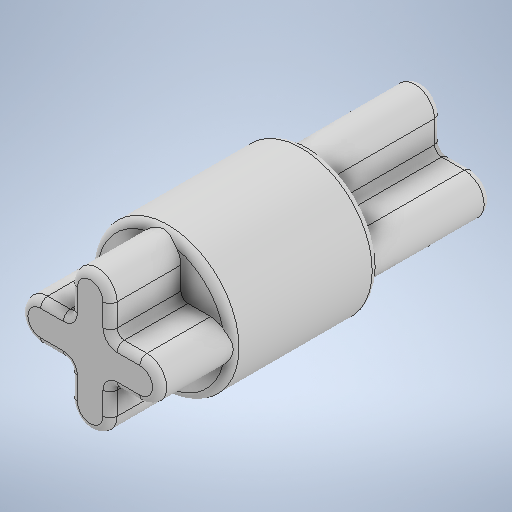
# Autodesk Inventor part: Axle
Saved by Autodesk Inventor 2025.2 (Build 292293000, 293)
## iProperties
Created: 2025-03-11
Part Number: Axle
Material: Generic
Document SubType Name: Modeling
Designer: eason
Density: 1 g/cm^3
Appearance: Default
Author: eason
Autodesk Inventor part; units mm, degrees
ref_plane "YZ Plane" through (0, 0, 0) normal (1, 0, 0) x (0, 1, 0)
ref_plane "XZ Plane" through (0, 0, 0) normal (0, 1, 0) x (-1, 0, 0)
ref_plane "XY Plane" through (0, 0, 0) normal (0, 0, 1) x (1, 0, 0)
sketch "Sketch1" plane through (0, 0, 0) normal (0, 0, 1) x (1, 0, 0)
  circle A0 centre (0, 0) radius 5
  circle A1 centre (0, 0) radius 2 construction
  circle A2 centre (0, 3.5) radius 1.5 construction
  line L0 (0, -7) -> (0, 7) projected
  circle A3 centre (0, 3.5) radius 1.4
  circle A4 centre (-3.5, 0) radius 1.4
  circle A5 centre (0, -3.5) radius 1.4
  circle A6 centre (3.5, 0) radius 1.4
  line L1 (-1.4, 3.5) -> (-1.4, 1.9)
  line L2 (-3.5, 1.4) -> (-1.9, 1.4)
  arc A7 (-1.9, 1.4) -> (-1.4, 1.9) centre (-1.9, 1.9) ccw
  line L3 (-1.4, -3.5) -> (-1.4, -1.9)
  arc A8 (-1.4, -1.9) -> (-1.9, -1.4) centre (-1.9, -1.9) ccw
  line L4 (-3.5, -1.4) -> (-1.9, -1.4)
  line L5 (3.5, -1.4) -> (1.9, -1.4)
  arc A9 (1.9, -1.4) -> (1.4, -1.9) centre (1.9, -1.9) ccw
  line L6 (1.4, -3.5) -> (1.4, -1.9)
  line L7 (1.4, 3.5) -> (1.4, 1.9)
  arc A10 (1.4, 1.9) -> (1.9, 1.4) centre (1.9, 1.9) ccw
  line L8 (3.5, 1.4) -> (1.9, 1.4)
  point P0 (1.4, 3.5)
  dimension "d0" = 10
  dimension "d2" = 0.1
  dimension "d5" = 360
  dimension "d14" = 3
  dimension "d15" = 0.5
  dimension "d18" = 360
  constraints: 16 end point, 9 centre point, 8 point on circle, 4 tangent, 3 coincident, 2 horizontal, 2 vertical, 1 perpendicular, 1 point on line, 48 other
  measures "d0" diameter of A0
  measures "d14" radial gap between concentric circles of A0 A1
  measures "d15" radius of A7
extrude "Extrusion1" add sketch "Sketch1" along normal blind 10.4
extrude "Extrusion2" add sketch "Sketch1" against normal blind 8 contours A3 L0 | L0 A3 | A5 L0 | L0 A5 | A3 L7 A10 L8 A6 L5 A9 L6 A5 L0 | L0 A5 L3 A8 L4 A4 L2 A7 L1 A3 | A6 | A4
sketch "Sketch3" plane through (0, 0, 10.4) normal (0, 0, 1) x (1, 0, 0)
  line L0 (3.5, 1.4) -> (1.9, 1.4) projected
  arc A0 (1.4, 1.9) -> (1.9, 1.4) centre (1.9, 1.9) ccw projected
  line L1 (1.4, 1.9) -> (1.4, 3.5) projected
  arc A1 (1.4, 3.5) -> (-1.4, 3.5) centre (0, 3.5) ccw projected
  line L2 (-1.4, 3.5) -> (-1.4, 1.9) projected
  arc A2 (-1.9, 1.4) -> (-1.4, 1.9) centre (-1.9, 1.9) ccw projected
  line L3 (-1.9, 1.4) -> (-3.5, 1.4) projected
  arc A3 (-3.5, 1.4) -> (-3.5, -1.4) centre (-3.5, 0) ccw projected
  line L4 (-3.5, -1.4) -> (-1.9, -1.4) projected
  arc A4 (-1.4, -1.9) -> (-1.9, -1.4) centre (-1.9, -1.9) ccw projected
  line L5 (-1.4, -1.9) -> (-1.4, -3.5) projected
  arc A5 (-1.4, -3.5) -> (1.4, -3.5) centre (0, -3.5) ccw projected
  line L6 (1.4, -3.5) -> (1.4, -1.9) projected
  arc A6 (1.9, -1.4) -> (1.4, -1.9) centre (1.9, -1.9) ccw projected
  line L7 (1.9, -1.4) -> (3.5, -1.4) projected
  arc A7 (3.5, -1.4) -> (3.5, 1.4) centre (3.5, 0) ccw projected
  circle A8 centre (0, 0) radius 5 projected
extrude "Extrusion4" add sketch "Sketch3" along normal blind 5 contours A7 L7 A6 L6 A5 L5 A4 L4 A3 L3 A2 L2 A1 L1 A0 L0
fillet "Fillet2" radius 0.5 34 edges at (-4.9, 0, -8) (-2.7, 1.4, -8) (-1.5464, 1.5464, -8) (-1.4, 2.7, -8) (0, 4.9, -8) (1.4, 2.7, -8) (1.5464, 1.5464, -8) (2.7, 1.4, -8) (4.9, 0, -8) (2.7, -1.4, -8) (1.5464, -1.5464, -8) (1.4, -2.7, -8) (0, -4.9, -8) (-1.4, -2.7, -8) (-1.5464, -1.5464, -8) (-2.7, -1.4, -8) (-2.7, -1.4, 15.4) (-1.5464, -1.5464, 15.4) (-1.4, -2.7, 15.4) (0, -4.9, 15.4) (1.4, -2.7, 15.4) (1.5464, -1.5464, 15.4) (2.7, -1.4, 15.4) (4.9, 0, 15.4) (2.7, 1.4, 15.4) (1.5464, 1.5464, 15.4) (1.4, 2.7, 15.4) (0, 4.9, 15.4) (-1.4, 2.7, 15.4) (-1.5464, 1.5464, 15.4) (-2.7, 1.4, 15.4) (-4.9, 0, 15.4) (-5, 0, 0) (-5, 0, 10.4)
body "Solid1"
